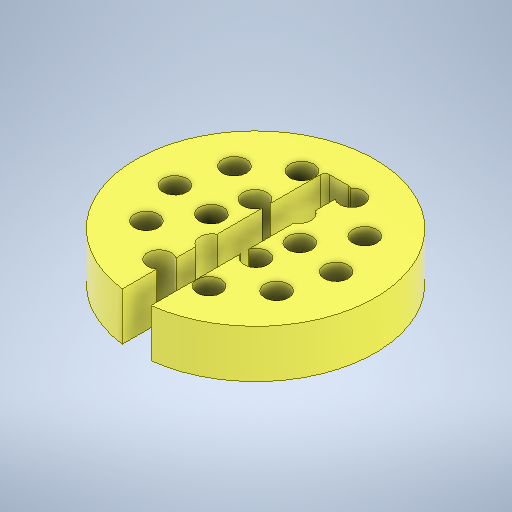
# Autodesk Inventor part: Filter_1
Saved by Autodesk Inventor 2025.2 (Build 292293000, 293)
## iProperties
Created: 2025-05-24
Part Number: Filter_1
Material: Steel
Document SubType Name: Modeling
Designer: Musa Gamal
Density: 7.85 g/cm^3
Appearance: Smooth - Yellow
Author: Musa Gamal
Autodesk Inventor part; units mm, degrees
ref_plane "YZ Plane" through (0, 0, 0) normal (1, 0, 0) x (0, 1, 0)
ref_plane "XZ Plane" through (0, 0, 0) normal (0, 1, 0) x (-1, 0, 0)
ref_plane "XY Plane" through (0, 0, 0) normal (0, 0, 1) x (1, 0, 0)
sketch "Sketch1" plane through (0, 0, 0) normal (0, 1, 0) x (-1, 0, 0)
  circle A0 centre (0, 0) radius 50
  circle A1 centre (10.7155, -10.4966) radius 5
  circle A2 centre (14.4481, 4.0316) radius 5
  circle A3 centre (3.7326, 14.5282) radius 5
  circle A4 centre (-10.7155, 10.4966) radius 5
  circle A5 centre (-14.4481, -4.0316) radius 5
  circle A6 centre (-3.7326, -14.5282) radius 5
  circle A7 centre (26.971, -18.1333) radius 5
  circle A8 centre (32.4785, 1.183) radius 5
  circle A9 centre (25.5803, 20.0474) radius 5
  circle A10 centre (8.9113, 31.2544) radius 5
  circle A11 centre (-11.1615, 30.5233) radius 5
  circle A12 centre (-26.971, 18.1333) radius 5
  circle A13 centre (-32.4785, -1.183) radius 5
  circle A14 centre (-25.5803, -20.0474) radius 5
  circle A15 centre (-8.9113, -31.2544) radius 5
  circle A16 centre (11.1615, -30.5233) radius 5
  dimension "d0" = 100
  dimension "d4" = 10
  dimension "d7" = 360
  dimension "d10" = 10
  dimension "d13" = 360
  constraints: 17 centre point, 1 coincident, 34 other
  measures "d0" diameter of A0
  measures "d4" diameter of A1
  measures "d10" diameter of A7
extrude "Extrusion1" add sketch "Sketch1" along normal blind 20
sketch "Sketch3" plane through (0, 20, 0) normal (0, 1, 0) x (1, 0, 0)
  line L0 (-6, 33) -> (-6, -55)
  line L1 (6, 33) -> (6, -55.679)
  line L2 (-4, 35) -> (4, 35)
  arc A0 (-4, 35) -> (-6, 33) centre (-4, 33) ccw
  arc A1 (6, 33) -> (4, 35) centre (4, 33) ccw
  circle A2 centre (0, 0) radius 50 projected
  circle A3 centre (-11.1615, 30.5233) radius 5 projected
  circle A4 centre (8.9113, 31.2544) radius 5 projected
  circle A5 centre (25.5803, 20.0474) radius 5 projected
  circle A6 centre (32.4785, 1.183) radius 5 projected
  circle A7 centre (26.971, -18.1333) radius 5 projected
  circle A8 centre (11.1615, -30.5233) radius 5 projected
  circle A9 centre (-8.9113, -31.2544) radius 5 projected
  circle A10 centre (-25.5803, -20.0474) radius 5 projected
  circle A11 centre (-32.4785, -1.183) radius 5 projected
  circle A12 centre (-26.971, 18.1333) radius 5 projected
  circle A13 centre (3.7326, 14.5282) radius 5 projected
  circle A14 centre (14.4481, 4.0316) radius 5 projected
  circle A15 centre (10.7155, -10.4966) radius 5 projected
  circle A16 centre (-3.7326, -14.5282) radius 5 projected
  circle A17 centre (-14.4481, -4.0316) radius 5 projected
  circle A18 centre (-10.7155, 10.4966) radius 5 projected
  point P0 (-6, 35)
  point P1 (0, 10)
  point P2 (-6, -10.0719)
  point P3 (-6, -18.9845)
  point P4 (-6, -49.6387)
  point P5 (6, -49.6387)
  point P6 (-6, -27.1894)
  point P7 (-6, -35.3194)
  point P8 (6, -12.1592)
  point P9 (6, -8.834)
  point P10 (0, 35)
  dimension "d26" = 6
  dimension "d27" = 90
  dimension "d28" = 12
  dimension "d29" = 2
  dimension "d30" = 2
  dimension "d34" = 35
  constraints: 6 end point, 4 point on circle, 4 tangent, 2 centre point, 2 point on line, 1 horizontal, 1 midpoint, 1 parallel, 1 vertical
  measures "d26" distance from line of point (0, 0) L0
  measures "d27" distance of point (-6, 35) L0.end
  measures "d28" distance between parallel lines of L0 L1
  measures "d29" radius of A0
  measures "d30" radius of A1
  measures "d34" distance of point (0, 0) point (0, 35)
extrude "Extrusion3" cut sketch "Sketch3" against normal through all contours A0 L2 A1 A4 L1 A13 A15 A2 L0 A9 A16 A18 | A18 L0 | L0 A18 | A16 L0 | L0 A16 | A4 L1 A1 | A1 L1 A4 | A9 L0 | L0 A9 | A13 L1 | L1 A13 | A15 L1 | L1 A15 | A3 | A5 | A6 | A7 | A8 | A10 | A11 | A12 | A14 | A17 picked at (2.6962, -31.0174)
body "Solid1"
